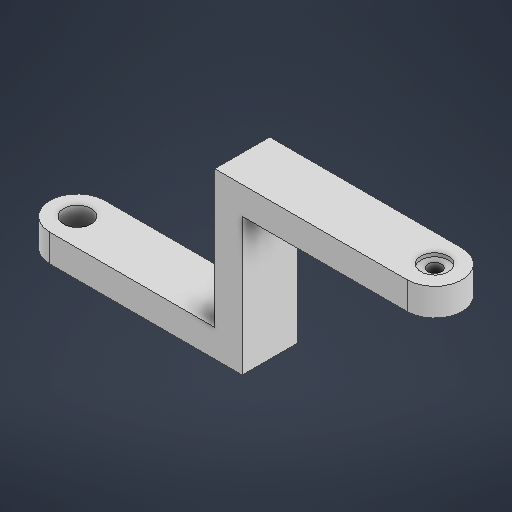
# Autodesk Inventor part: Part2
Saved by Autodesk Inventor 2026 (Build 300175000, 175)
## iProperties
Created: 2025-05-07
Part Number: Part2
Material: Generic
Document SubType Name: Modeling
Designer: Ritul Kumari
Density: 1 g/cm^3
Appearance: Default
Author: Ritul Kumari
Autodesk Inventor part; units mm, degrees
ref_plane "YZ Plane" through (0, 0, 0) normal (1, 0, 0) x (0, 1, 0)
ref_plane "XZ Plane" through (0, 0, 0) normal (0, 1, 0) x (-1, 0, 0)
ref_plane "XY Plane" through (0, 0, 0) normal (0, 0, 1) x (1, 0, 0)
sketch "Sketch1" plane through (0, 0, 0) normal (0, 0, 1) x (1, 0, 0)
  line L0 (0, 0) -> (-101.6, 0)
  line L1 (-101.6, 0) -> (-101.6, 12.7)
  line L2 (-101.6, 12.7) -> (-12.7, 12.7)
  line L3 (0, 12.7) -> (0, 0)
  line L4 (0, 0) -> (-12.7, 0)
  line L5 (-12.7, 12.7) -> (-12.7, 76.2)
  line L6 (-12.7, 76.2) -> (88.9, 76.2)
  line L7 (88.9, 76.2) -> (88.9, 63.5)
  line L8 (88.9, 63.5) -> (0, 63.5)
  line L9 (0, 63.5) -> (0, 12.7)
  dimension "d0" = 101.6
  dimension "d4" = 12.7
  dimension "d5" = 12.7
  dimension "d6" = 12.7
  dimension "d7" = 76.2
  dimension "d8" = 101.6
  dimension "d9" = 12.7
  dimension "d10" = 88.9
  constraints: 20 end point, 5 perpendicular, 2 horizontal, 1 point on line, 1 vertical
  measures "d0" distance of L0.start L0.end
  measures "d4" distance of L0.end L1.end
  measures "d5" distance of L3.start L0.start
  measures "d6" distance of L0.start L4.end
  measures "d7" distance of L4.end L5.end
  measures "d8" distance of L5.end L6.end
  measures "d9" distance of L6.end L7.end
  measures "d10" distance of L7.end L8.end
extrude "Extrusion1" add sketch "Sketch1" along normal mid plane 25.4
fillet "Fillet1" radius 12.7 1 edges at (88.9, 69.85, -12.7)
fillet "Fillet2" radius 12.7 1 edges at (88.9, 69.85, 12.7)
fillet "Fillet3" radius 12.7 1 edges at (-101.6, 6.35, -12.7)
fillet "Fillet4" radius 12.7 1 edges at (-101.6, 6.35, 12.7)
sketch "Sketch2" plane through (-12.7, 12.7, 12.7) normal (0, 1, 0) x (1, 0, 0)
  arc A0 (-76.2, 25.4) -> (-76.2, 0) centre (-76.2, 12.7) ccw projected
  circle A1 centre (-76.2, 12.7) radius 6.35
  point P0 (12.7, 12.7)
  dimension "d17" = 12.7
  constraints: 1 centre point, 1 coincident
  measures "d17" diameter of A1
extrude "Extrusion2" cut sketch "Sketch2" against normal blind 25.4
sketch "Sketch3" plane through (-12.7, 76.2, 12.7) normal (0, 1, 0) x (1, 0, 0)
  arc A0 (88.9, 0) -> (88.9, 25.4) centre (88.9, 12.7) ccw projected
  point P0 (12.7, 12.7)
  constraints: 1 coincident
hole "Hole1" at (76.2, 76.2, 0) direction (0, -1, 0) diameter 6.35 end through all counterbore diameter 12.7 counterbore depth 1.5875
